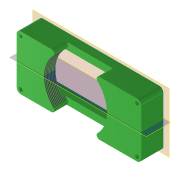
# Autodesk Inventor part: ESP32ParasiteMicroscope_middle_v0
Saved by Autodesk Inventor 2022 (Build 260153000, 153)
## iProperties
Created: 2022-02-02
Part Number: ESP32ParasiteMicroscope_middle_v0
Material: Generisch
Document SubType Name: Modeling
Designer: diederichbenedict
Density: 1 g/cm^3
Appearance: Glatt - Waldgrün
Author: diederichbenedict
Autodesk Inventor part; units mm, degrees
ref_plane "YZ Plane" through (0, 0, 0) normal (1, 0, 0) x (0, 1, 0)
ref_plane "Arbeitsebene1" through (0, 0, 0) normal (0, 0, 1) x (1, 0, 0)
sketch "Skizze1" plane through (0, 0, 0) normal (0, 0, 1) x (1, 0, 0)
  circle A0 centre (57.3299, 16.4874) radius 1.4 projected
  circle A1 centre (-25.745, -16.4874) radius 1.4 projected
  circle A2 centre (57.3299, -16.4874) radius 1.4 projected
  circle A3 centre (-25.745, 16.4874) radius 1.15 projected
  circle A4 centre (9.875, 11.6896) radius 0.65 projected
  circle A5 centre (9.875, -11.3104) radius 0.65 projected
  circle A6 centre (14.955, 11.6896) radius 0.65 projected
  circle A7 centre (14.955, -11.3104) radius 0.65 projected
  circle A8 centre (25.115, 11.6896) radius 0.65 projected
  circle A9 centre (25.115, -11.3104) radius 0.65 projected
  circle A10 centre (30.195, 11.6896) radius 0.65 projected
  circle A11 centre (30.195, -11.3104) radius 0.65 projected
  circle A12 centre (-2.825, -11.3104) radius 0.65 projected
  circle A13 centre (-2.825, 11.6896) radius 0.65 projected
  circle A14 centre (-0.285, -11.3104) radius 0.65 projected
  circle A15 centre (-0.285, 11.6896) radius 0.65 projected
  circle A16 centre (2.255, -11.3104) radius 0.65 projected
  circle A17 centre (2.255, 11.6896) radius 0.65 projected
  circle A18 centre (4.795, -11.3104) radius 0.65 projected
  circle A19 centre (4.795, 11.6896) radius 0.65 projected
  circle A20 centre (27.655, -11.3104) radius 0.65 projected
  circle A21 centre (27.655, 11.6896) radius 0.65 projected
  circle A22 centre (22.575, -11.3104) radius 0.65 projected
  circle A23 centre (22.575, 11.6896) radius 0.65 projected
  circle A24 centre (17.495, -11.3104) radius 0.65 projected
  circle A25 centre (17.495, 11.6896) radius 0.65 projected
  circle A26 centre (12.415, -11.3104) radius 0.65 projected
  circle A27 centre (12.415, 11.6896) radius 0.65 projected
  circle A28 centre (7.335, -11.3104) radius 0.65 projected
  circle A29 centre (7.335, 11.6896) radius 0.65 projected
  circle A30 centre (20.035, 11.6896) radius 0.65 projected
  circle A31 centre (20.035, -11.3104) radius 0.65 projected
  arc A32 (-28.745, -16.4874) -> (-25.745, -19.4874) centre (-25.745, -16.4874) ccw projected
  line L0 (57.3299, -19.4874) -> (-25.745, -19.4874) projected
  arc A33 (57.3299, -19.4874) -> (60.3299, -16.4874) centre (57.3299, -16.4874) ccw projected
  line L1 (60.3299, 16.4874) -> (60.3299, -16.4874) projected
  arc A34 (60.3299, 16.4874) -> (57.3299, 19.4874) centre (57.3299, 16.4874) ccw projected
  line L2 (-25.745, 19.4874) -> (57.3299, 19.4874) projected
  arc A35 (-25.745, 19.4874) -> (-28.745, 16.4874) centre (-25.745, 16.4874) ccw projected
  line L3 (-28.745, -16.4874) -> (-28.745, 16.4874) projected
  line L4 (55.3299, 14.4874) -> (55.3299, -14.4874)
  line L5 (55.3299, -14.4874) -> (-23.745, -14.4874)
  line L6 (-23.745, -14.4874) -> (-23.745, 14.4874)
  line L7 (-23.745, 14.4874) -> (55.3299, 14.4874)
  point P0 (0, 0)
  dimension "d0" = 5
  constraints: 8 end point, 3 other
  measures "d0" distance between parallel lines of L2 L7
ref_plane "Arbeitsebene2" through (-3.9015, -6.25, 7.6898) normal (0, 0, 1) x (1, 0, 0)
extrude "Extrusion1" add sketch "Skizze1" along normal up to surface (7.6898 mm away) contours L3 A35 L2 A34 L1 A33 L0 A32
sketch "Skizze2" plane through (-25.745, -19.4874, 7.6898) normal (0, 0, 1) x (1, 0, 0)
  circle A0 centre (83.0749, 35.9749) radius 1.4 projected
  circle A1 centre (0, 3) radius 1.4 projected
  circle A2 centre (83.0749, 3) radius 1.4 projected
  circle A3 centre (0, 35.9749) radius 1.15 projected
  line L0 (81.0749, 33.9749) -> (2, 33.9749) projected
  line L1 (81.0749, 5) -> (81.0749, 33.9749) projected
  line L2 (2, 5) -> (81.0749, 5) projected
  line L3 (2, 33.9749) -> (2, 5) projected
  arc A4 (0, 38.9749) -> (-3, 35.9749) centre (0, 35.9749) ccw projected
  line L4 (-3, 3) -> (-3, 35.9749) projected
  arc A5 (-3, 3) -> (0, 0) centre (0, 3) ccw projected
  line L5 (83.0749, 0) -> (0, 0) projected
  arc A6 (83.0749, 0) -> (86.0749, 3) centre (83.0749, 3) ccw projected
  line L6 (86.0749, 35.9749) -> (86.0749, 3) projected
  arc A7 (86.0749, 35.9749) -> (83.0749, 38.9749) centre (83.0749, 35.9749) ccw projected
  line L7 (0, 38.9749) -> (83.0749, 38.9749) projected
  circle A8 centre (39.0935, 19.4874) radius 3.8655 projected
  line L8 (43.0093, 18.0044) -> (43.0093, 15.5716) projected
  line L9 (43.0093, 15.322) -> (35.1777, 15.322) projected
  line L10 (35.1777, 23.4033) -> (37.6105, 23.4033) projected
  line L11 (34.9281, 15.5716) -> (34.9281, 23.4033) projected
  line L12 (43.3435, 23.4874) -> (43.3435, 15.4874) projected
  line L13 (35.0935, 23.7374) -> (43.0935, 23.7374) projected
  line L14 (34.9281, 15.5716) -> (34.9281, 23.4033) projected
  line L15 (34.9935, 15.3874) -> (43.1935, 15.3874)
  line L16 (43.1935, 15.3874) -> (43.1935, 23.5874)
  line L17 (43.1935, 23.5874) -> (34.9935, 23.5874)
  line L18 (34.9935, 23.5874) -> (34.9935, 15.3874)
  line L19 (34.9935, 15.3874) -> (43.1935, 23.5874) construction
  line L20 (43.1935, 15.3874) -> (34.9935, 23.5874) construction
  point P0 (25.745, 19.4874)
  dimension "d3" = 8.2
  dimension "d4" = 8.2
  constraints: 12 end point, 2 midpoint, 2 parallel, 1 horizontal, 1 perpendicular
  measures "d3" distance of L17.end L16.end
  measures "d4" distance of L16.end L15.end
extrude "Extrusion2" add sketch "Skizze2" along normal blind 2.2 contours L1 L2 L3 L0 | L7 A7 L6 A6 L5 A5 L4 A4
ref_plane "Arbeitsebene3" through (-21.9576, -12.7, 16.9028) normal (0, 0, -1) x (0, 1, 0)
sketch "Skizze3" plane through (-25.745, -19.4874, 9.8898) normal (0, 0, 1) x (1, 0, 0)
  line L0 (83.0749, 38.9749) -> (0, 38.9749) projected
  arc A0 (0, 38.9749) -> (-3, 35.9749) centre (0, 35.9749) ccw projected
  line L1 (-3, 35.9749) -> (-3, 3) projected
  arc A1 (-3, 3) -> (0, 0) centre (0, 3) ccw projected
  line L2 (0, 0) -> (83.0749, 0) projected
  arc A2 (83.0749, 0) -> (86.0749, 3) centre (83.0749, 3) ccw projected
  line L3 (86.0749, 3) -> (86.0749, 35.9749) projected
  arc A3 (86.0749, 35.9749) -> (83.0749, 38.9749) centre (83.0749, 35.9749) ccw projected
  line L4 (34.9935, 15.3874) -> (34.9935, 23.5874) projected
  line L5 (34.9935, 23.5874) -> (43.1935, 23.5874) projected
  line L6 (43.1935, 23.5874) -> (43.1935, 15.3874) projected
  line L7 (43.1935, 15.3874) -> (34.9935, 15.3874) projected
  circle A4 centre (0, 35.9749) radius 1.15 projected
  circle A5 centre (83.0749, 3) radius 1.4 projected
  circle A6 centre (0, 3) radius 1.4 projected
  circle A7 centre (83.0749, 35.9749) radius 1.4 projected
  circle A8 centre (39.0935, 19.4874) radius 3.6158 projected
  circle A9 centre (39.0935, 19.4874) radius 3.475
  point P0 (25.745, 19.4874)
  dimension "d7" = 6.95
  constraints: 1 centre point, 1 coincident
  measures "d7" diameter of A9
extrude "Extrusion3" add sketch "Skizze3" along normal blind 6 contours A3 L3 A2 L2 A1 L1 A0 L0 | L4 L5 L6 L7
sketch "Skizze4" plane through (-25.745, 19.4874, 15.8898) normal (0, 0, 1) x (1, 0, 0)
  circle A0 centre (39.0935, -19.4874) radius 3.6158 projected
  circle A1 centre (39.0935, -19.4874) radius 22.5
  point P0 (25.745, -19.4874)
  dimension "d10" = 45
  constraints: 1 centre point, 1 coincident
  measures "d10" diameter of A1
extrude "Extrusion4" cut sketch "Skizze4" against normal blind 10
ref_plane "Arbeitsebene4" through (-25.745, 0, 0) normal (0, -1, 0) x (1, 0, 0)
fillet "Rundung1" radius 2 4 edges at (2.1017, -19.4874, 10.8898) (24.5952, -19.4874, 10.8898) (2.1017, 19.4874, 10.8898) (24.5952, 19.4874, 10.8898)
thread "Gewinde1" size "M45x1" class "6H" standard "ANSI Metric M Profile" full length
